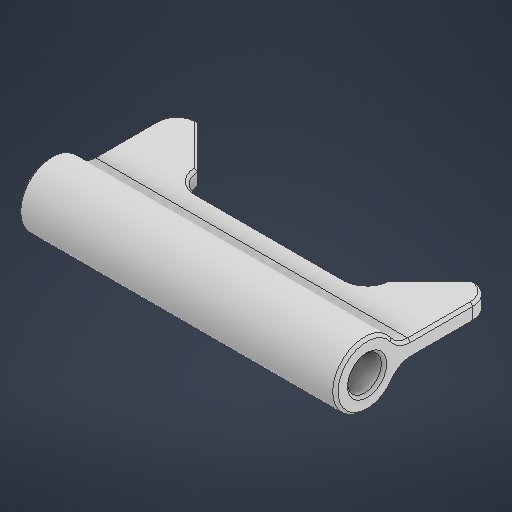
# Autodesk Inventor part: CoinLockUpperRow2
Saved by Autodesk Inventor 2026.3 (Build 303398000, 398)
## iProperties
Created: 2026-05-05
Part Number: CoinLockUpperRow2
Material: Generic
Document SubType Name: Modeling
Designer: frede
Density: 1 g/cm^3
Appearance: Default
Author: frede
Autodesk Inventor part; units mm, degrees
ref_plane "YZ Plane" through (0, 0, 0) normal (1, 0, 0) x (0, 1, 0)
ref_plane "XZ Plane" through (0, 0, 0) normal (0, 1, 0) x (-1, 0, 0)
ref_plane "XY Plane" through (0, 0, 0) normal (0, 0, 1) x (1, 0, 0)
sketch "Sketch3" plane through (0, 0, 0) normal (1, 0, 0) x (0, 1, 0)
  circle A0 centre (0, 0) radius 1.6
  arc A1 (1.725, -2.4545) -> (-1.6531, -2.5034) centre (0, 0) ccw
  line L0 (-0.7552, -4.1724) -> (-0.7552, -12)
  line L1 (-0.7552, -12) -> (0.875, -12)
  line L2 (0.875, -12) -> (0.875, -4.0908)
  arc A2 (1.725, -2.4545) -> (0.875, -4.0908) centre (2.875, -4.0908) ccw
  arc A3 (-0.7552, -4.1724) -> (-1.6531, -2.5034) centre (-2.7552, -4.1724) ccw
  dimension "d4" = 3.2
  dimension "d5" = 6
  dimension "d7" = 2
  dimension "d33" = 12
  constraints: 6 end point, 6 point on circle, 4 centre point, 4 tangent, 2 coincident, 1 equal radius, 1 parallel
  measures "d4" diameter of A0
  measures "d5" diameter of A1
  measures "d7" radius of A2
  measures "d33" distance from line of point (0, 0) L1
extrude "Extrusion2" add sketch "Sketch3" along normal blind 30
sketch "Sketch5" plane through (0, 0.875, -4.0908) normal (0, 1, 0) x (1, 0, 0)
  line L0 (0, 7.9092) -> (30, 7.9092) projected
  line L1 (6, 7.9092) -> (24, 7.9092)
  line L2 (24, 7.9092) -> (24, 1.9092)
  line L3 (24, 1.9092) -> (6, 1.9092)
  line L4 (6, 1.9092) -> (6, 7.9092)
  line L5 (0, 7.9092) -> (0, 0) projected
  point P0 (0, -4.0908)
  dimension "d18" = 6
  dimension "d19" = 30
  dimension "d20" = 6
  dimension "d21" = 18
  constraints: 8 end point, 2 parallel, 1 horizontal, 1 perpendicular, 1 point on line
  measures "d18" distance of L1.end L2.end
  measures "d19" distance of L0.start L0.end
  measures "d20" distance between parallel lines of L5 L4
  measures "d21" distance between parallel lines of L2 L4
extrude "Extrusion3" cut sketch "Sketch5" along normal blind 0.5 and the other way blind 2
chamfer "Chamfer3" distance 4 angle 45 2 edges at (6, 0.0599, -12) (24, 0.0599, -12)
fillet "Fillet1" radius 2 4 edges at (30, 0.0599, -12) (0, 0.0599, -12) (24, 0.0599, -6) (6, 0.0599, -6)
chamfer "Chamfer2" distance 0.25 angle 45 28 edges at (6, 0.875, -7.9998) (6.5856, 0.875, -6.5856) (23.4144, 0.875, -6.5856) (24, 0.875, -7.9998) (29.4144, 0.875, -11.4144) (30, 0.875, -7.0456) (30, 1.1002, -3.1688) (30, -0.0435, 2.9997) (30, -0.9939, -3.2248) (30, -0.7552, -7.0865) (29.4144, -0.7552, -11.4144) (23.4144, -0.7552, -6.5856) (24, -0.7552, -7.9997) (6, -0.7552, -7.9998) (6.5856, -0.7552, -6.5856) (0.5856, -0.7552, -11.4144) (0, -0.7552, -7.0865) (0, -0.9939, -3.2248) (0, -0.0435, 2.9997) (0, 1.1002, -3.1688) (0, 0.875, -7.0456) (0.5856, 0.875, -11.4144) (30, -1.6, 0) (0, -1.6, 0) (26, 0.875, -10) (26, -0.7552, -10) (4, 0.875, -10) (4, -0.7552, -10)
equation "\"d20\" = -0.5 * d21 + 0.5 * d19"
body "Solid2"
